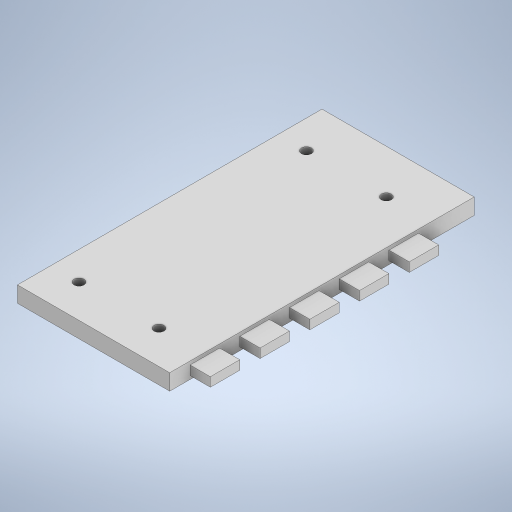
# Autodesk Inventor part: pca
Saved by Autodesk Inventor 2024.3 (Build 283343000, 343)
## iProperties
Created: 2025-10-13
Part Number: pca
Material: Generic
Document SubType Name: Modeling
Designer: jscme
Density: 1 g/cm^3
Appearance: Default
Author: jscme
Autodesk Inventor part; units mm, degrees
ref_plane "YZ Plane" through (0, 0, 0) normal (1, 0, 0) x (0, 1, 0)
ref_plane "XZ Plane" through (0, 0, 0) normal (0, 1, 0) x (-1, 0, 0)
ref_plane "XY Plane" through (0, 0, 0) normal (0, 0, 1) x (1, 0, 0)
sketch "Sketch1" plane through (0, 0, 0) normal (0, 1, 0) x (-1, 0, 0)
  line L0 (19.05, 38.1) -> (-19.05, 38.1)
  line L1 (-19.05, 38.1) -> (-19.05, -38.1)
  line L2 (-19.05, -38.1) -> (19.05, -38.1)
  line L3 (19.05, -38.1) -> (19.05, 38.1)
  point P0 (0, 0)
  point P1 (19.05, 0)
  point P2 (0, -38.1)
  dimension "d0" = 76.2
  dimension "d1" = 38.1
  constraints: 8 end point, 2 midpoint, 2 parallel, 1 horizontal, 1 horizontal alignment, 1 perpendicular, 1 vertical alignment
  measures "d0" distance of L2.end L0.start
  measures "d1" distance between parallel lines of L1 L3
extrude "Extrusion1" add sketch "Sketch1" along normal blind 4
sketch "Sketch2" plane through (19.05, 0, 38.1) normal (1, 0, 0) x (0, 0, -1)
  line L0 (5.08, 3.143) -> (12.446, 3.143)
  line L1 (12.446, 3.143) -> (12.446, 0.857)
  line L2 (12.446, 0.857) -> (5.08, 0.857)
  line L3 (5.08, 0.857) -> (5.08, 3.143)
  line L4 (0, 0) -> (0, 4) projected
  line L5 (0, 4) -> (76.2, 4) projected
  line L6 (17.526, 3.143) -> (24.892, 3.143)
  line L7 (24.892, 3.143) -> (24.892, 0.857)
  line L8 (24.892, 0.857) -> (17.526, 0.857)
  line L9 (17.526, 0.857) -> (17.526, 3.143)
  line L10 (29.972, 3.143) -> (37.338, 3.143)
  line L11 (37.338, 3.143) -> (37.338, 0.857)
  line L12 (37.338, 0.857) -> (29.972, 0.857)
  line L13 (29.972, 0.857) -> (29.972, 3.143)
  line L14 (42.418, 3.143) -> (49.784, 3.143)
  line L15 (49.784, 3.143) -> (49.784, 0.857)
  line L16 (49.784, 0.857) -> (42.418, 0.857)
  line L17 (42.418, 0.857) -> (42.418, 3.143)
  line L18 (54.864, 3.143) -> (62.23, 3.143)
  line L19 (62.23, 3.143) -> (62.23, 0.857)
  line L20 (62.23, 0.857) -> (54.864, 0.857)
  line L21 (54.864, 0.857) -> (54.864, 3.143)
  point P0 (38.1, 0)
  point P1 (5.08, 2)
  point P2 (0, 2)
  point P3 (17.526, 2)
  point P4 (0, 2)
  point P5 (29.972, 2)
  point P6 (0, 2)
  point P7 (42.418, 2)
  point P8 (0, 2)
  dimension "d4" = 5.08
  dimension "d5" = 7.366
  dimension "d6" = 2.286
  dimension "d8" = 5.08
  dimension "d9" = 7.366
  dimension "d10" = 2.286
  dimension "d11" = 7.366
  dimension "d12" = 2.286
  dimension "d13" = 5.08
  dimension "d14" = 7.366
  dimension "d15" = 2.286
  dimension "d16" = 5.08
  dimension "d18" = 7.366
  dimension "d19" = 5.08
  constraints: 40 end point, 10 parallel, 8 midpoint, 5 horizontal, 5 perpendicular, 4 horizontal alignment, 2 point on line
  measures "d4" distance between parallel lines of L4 L3
  measures "d5" distance of L0.start L0.end
  measures "d6" distance of L0.end L1.end
  measures "d8" distance between parallel lines of L1 L9
  measures "d9" distance of L7.end L8.end
  measures "d10" distance between parallel lines of L8 L6
  measures "d11" distance of L11.end L12.end
  measures "d12" distance between parallel lines of L12 L10
  measures "d13" distance between parallel lines of L7 L13
  measures "d14" distance of L15.end L16.end
  measures "d15" distance between parallel lines of L16 L14
  measures "d16" distance between parallel lines of L11 L17
  measures "d18" distance of L19.end L20.end
  measures "d19" distance from line of L15 L20.end
extrude "Extrusion2" add sketch "Sketch2" along normal blind 5.08
sketch "Sketch4" plane through (0, 4, 0) normal (0, 1, 0) x (1, 0, 0)
  circle A0 centre (8.05, 27.1) radius 1.27
  line L0 (19.05, -38.1) -> (19.05, 38.1) projected
  line L1 (19.05, 38.1) -> (-19.05, 38.1) projected
  circle A1 centre (-11.95, 27.1) radius 1.27
  line L2 (-19.05, 38.1) -> (-19.05, -38.1) projected
  circle A2 centre (8.05, -29.796) radius 1.27
  circle A3 centre (-11.95, -29.796) radius 1.27
  line L3 (-19.05, -38.1) -> (19.05, -38.1) projected
  point P0 (0, 0)
  dimension "d27" = 11
  dimension "d28" = 11
  dimension "d31" = 2.54
  dimension "d32" = 2.54
  dimension "d37" = 2.54
  dimension "d38" = 2.54
  dimension "d41" = 20
  dimension "d42" = 56.896
  dimension "d43" = 56.896
  constraints: 4 centre point, 2 vertical alignment
  measures "d27" distance from line of L0 A0.centre
  measures "d28" distance from line of L1 A0.centre
  measures "d31" diameter of A0
  measures "d32" diameter of A1
  measures "d37" diameter of A3
  measures "d38" diameter of A2
  measures "d41" distance of A1.centre A0.centre
  measures "d42" distance of A1.centre A3.centre
  measures "d43" distance of A0.centre A2.centre
extrude "Extrusion4" cut sketch "Sketch4" against normal blind 7.1628 contours A0 | A1 | A2 | A3
body "Solid1"
